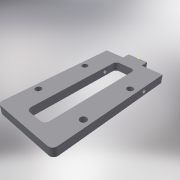
# Autodesk Inventor part: BallBalancing_MotorPlate
Saved by Autodesk Inventor 2016 (Build 200138000, 138)
## iProperties
Created: 2016-04-08
Part Number: BallBalancing_MotorPlate
Material: Generic
Document SubType Name: Modeling
Designer: Admin
Density: 1 g/cm^3
Appearance: Default
Author: Admin
Autodesk Inventor part; units mm, degrees
ref_plane "YZ Plane" through (0, 0, 0) normal (1, 0, 0) x (0, 1, 0)
ref_plane "XZ Plane" through (0, 0, 0) normal (0, 1, 0) x (-1, 0, 0)
ref_plane "XY Plane" through (0, 0, 0) normal (0, 0, 1) x (1, 0, 0)
sketch "Sketch1" plane through (0, 0, 0) normal (0, 0, 1) x (1, 0, 0)
  line L0 (-15, 0) -> (15, 0)
  line L1 (15, 0) -> (15, -60)
  line L2 (15, -60) -> (-15, -60)
  line L3 (-15, -60) -> (-15, 0)
  line L4 (-21, 0) -> (21, 0) projected
  line L5 (0, -72) -> (0, 12) projected
  point P0 (0, 0)
  dimension "d0" = 30
  dimension "d1" = 60
  dimension "d4" = 15
  constraints: 8 end point, 2 parallel, 1 collinear, 1 horizontal, 1 perpendicular
  measures "d0" distance of L0.start L0.end
  measures "d1" distance of L0.end L1.end
  measures "d4" distance between parallel lines of L1 L5
extrude "Extrusion1" add sketch "Sketch1" along normal blind 4
sketch "Sketch2" plane through (0, 0, 4) normal (0, 0, 1) x (1, 0, 0)
  line L0 (15, 0) -> (-15, 0) projected
  line L1 (-15, 0) -> (-15, -60) projected
  line L2 (-15, -60) -> (15, -60) projected
  line L3 (15, -60) -> (15, 0) projected
  line L4 (0, -72) -> (0, 12) projected
  circle A0 centre (-12, -21) radius 1.5
  circle A1 centre (-12, -45) radius 1.5
  circle A2 centre (12, -21) radius 1.5
  circle A3 centre (12, -45) radius 1.5
  line L5 (15, 0) -> (-15, 0) projected
  line L6 (15, -60) -> (15, 0) projected
  line L7 (4.7021, 0) -> (15, 0)
  line L8 (15, 0) -> (15, -4)
  line L9 (15, -4) -> (4.7021, -4)
  line L10 (4.7021, -4) -> (4.7021, 0)
  line L11 (-15, 0) -> (-15, -60) projected
  line L12 (-5.2979, 0) -> (-15, 0)
  line L13 (-15, 0) -> (-15, -4)
  line L14 (-15, -4) -> (-5.2979, -4)
  line L15 (-5.2979, -4) -> (-5.2979, 0)
  line L16 (-3, -9) -> (3, -9)
  line L17 (5, -11) -> (5, -53)
  line L18 (3, -55) -> (-3, -55)
  line L19 (-5, -53) -> (-5, -11)
  arc A4 (-3, -9) -> (-5, -11) centre (-3, -11) ccw
  arc A5 (5, -11) -> (3, -9) centre (3, -11) ccw
  arc A6 (3, -55) -> (5, -53) centre (3, -53) ccw
  arc A7 (-5, -53) -> (-3, -55) centre (-3, -53) ccw
  point P0 (0, 0)
  dimension "d5" = 3
  dimension "d6" = 12
  dimension "d7" = 3
  dimension "d8" = 12
  dimension "d9" = 24
  dimension "d10" = 15
  dimension "d13" = 4
  dimension "d14" = 10
  dimension "d15" = 5
  dimension "d16" = 10
  dimension "d18" = 5
  dimension "d19" = 2
  dimension "d28" = 10
  constraints: 24 end point, 8 centre point, 8 point on circle, 8 tangent, 6 parallel, 5 point on line, 3 equal radius, 3 horizontal, 3 perpendicular, 2 symmetric about line, 2 other
  measures "d5" diameter of A0
  measures "d6" distance from line of L4 A0.centre
  measures "d7" diameter of A1
  measures "d8" distance from line of L4 A1.centre
  measures "d9" distance of A0.centre A1.centre
  measures "d10" distance from line of L2 A1.centre
  measures "d13" distance between parallel lines of L12 L14
  measures "d14" distance between parallel lines of L10 L15
  measures "d15" distance between parallel lines of L2 L18
  measures "d16" distance between parallel lines of L3 L17
  measures "d18" distance between parallel lines of L14 L16
  measures "d19" radius of A4
  measures "d28" distance between parallel lines of L1 L19
extrude "Extrusion2" cut sketch "Sketch2" against normal blind 4 contours L3 L9 L10 L0 | L15 L14 L1 L0 | L16 A5 L17 A6 L18 L4 | L4 L18 A7 L19 A4 L16 | A0 | A1 | A2 | A3
sketch "Sketch3" plane through (0, 0, 4) normal (0, 0, 1) x (1, 0, 0)
  point P0 (0, 0)
fillet "Fillet1" radius 2 2 edges at (15, -60, 2) (-15, -60, 2)
sketch "Sketch4" plane through (4.7021, -4, 4) normal (1, 0, 0) x (0, 0, -1)
  line L0 (0, 0) -> (0, 4) projected
  line L1 (0, 0) -> (4, 0) projected
  line L2 (4, 4) -> (4, 0) projected
  line L3 (0, 4) -> (4, 4) projected
  line L4 (0, 0) -> (4, 0) projected
  line L5 (2, 0) -> (2, 4) construction
  line L6 (0, 4) -> (4, 4) projected
  circle A0 centre (2, 2) radius 1
  dimension "d21" = 2
  constraints: 3 midpoint, 2 end point, 1 centre point
  measures "d21" diameter of A0
extrude "Extrusion3" cut sketch "Sketch4" against normal through all contours A0
sketch "Sketch5" plane through (15, -4, 4) normal (1, 0, 0) x (0, 0, -1)
  line L0 (4, -54) -> (0, -54) projected
  line L1 (4, 0) -> (4, -54) projected
  line L2 (4, 0) -> (0, 0) projected
  line L3 (0, -54) -> (0, 0) projected
  circle A0 centre (2, 2) radius 1 projected
  circle A1 centre (2, 2) radius 1 projected
  line L4 (2, 2) -> (2, -25.9382) construction
  circle A2 centre (2, -12) radius 1
  point P0 (4, 4)
  dimension "d24" = 2
  dimension "d25" = 14
  constraints: 2 end point, 1 centre point, 1 point on line, 1 vertical
  measures "d24" diameter of A2
  measures "d25" distance of A0.centre A2.centre
extrude "Extrusion4" cut sketch "Sketch5" against normal through all contours A2
equation "\"d4\" = 0.5 * d0"
body "Solid1"
